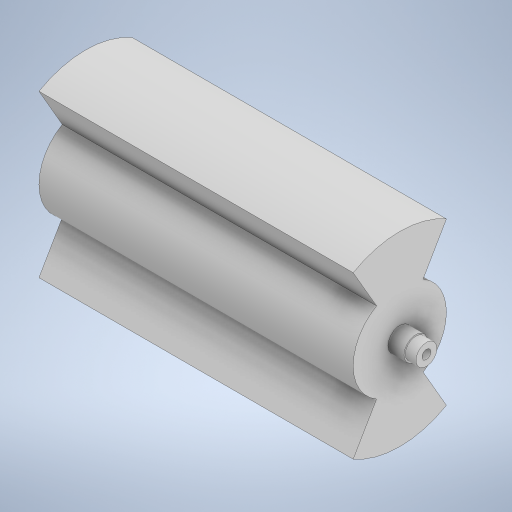
# Autodesk Inventor part: newDrum
Saved by Autodesk Inventor 2024.2 (Build 282272000, 272)
## iProperties
Created: 2024-02-27
Part Number: newDrum
Material: Generic
Document SubType Name: Modeling
Designer: jerem
Density: 1 g/cm^3
Appearance: Default
Author: jerem
## iProperties of the stored document newDrum_3DPrint.ipt
Created: 2024-02-27
Part Number: newDrum_3DPrint
Material: Generic
Document SubType Name: Modeling
Designer: jerem
Density: 1 g/cm^3
Appearance: Default
Author: jerem
Autodesk Inventor part; units mm, degrees
ref_plane "YZ Plane" through (0, 0, 0) normal (1, 0, 0) x (0, 1, 0)
ref_plane "XZ Plane" through (0, 0, 0) normal (0, 1, 0) x (-1, 0, 0)
ref_plane "XY Plane" through (0, 0, 0) normal (0, 0, 1) x (1, 0, 0)
sketch "Sketch1" plane through (0, 0, 0) normal (1, 0, 0) x (0, 1, 0)
  circle A0 centre (0, 0) radius 17.5
  dimension "d1" = 35
  constraints: 1 centre point
  measures "d1" diameter of A0
extrude "Extrusion1" add sketch "Sketch1" along normal blind 118
sketch "Sketch2" plane through (0, 0, 0) normal (-1, 0, 0) x (0, 0, 1)
  circle A0 centre (0, 0) radius 13.9
  dimension "d4" = 27.8
  constraints: 1 centre point, 1 coincident
  measures "d4" diameter of A0
extrude "Extrusion2" cut sketch "Sketch2" against normal blind 16
sketch "Sketch3" plane through (16, 0, 0) normal (-1, 0, 0) x (0, 0, 1)
  circle A0 centre (0, 0) radius 4.85
  dimension "d7" = 9.7
  constraints: 1 centre point, 1 coincident
  measures "d7" diameter of A0
extrude "Extrusion3" cut sketch "Sketch3" against normal blind 4.2
sketch "Sketch4" plane through (20.2, 0, 0) normal (-1, 0, 0) x (0, 0, 1)
  circle A0 centre (0, 0) radius 1.7
  dimension "d10" = 3.4
  constraints: 1 centre point, 1 coincident
  measures "d10" diameter of A0
extrude "Extrusion4" cut sketch "Sketch4" against normal blind 10
sketch "Sketch9" plane through (0, 0, 0) normal (1, 0, 0) x (0, 1, 0)
  circle A0 centre (0, 0) radius 1.7 construction
  circle A1 centre (0, 0) radius 35 construction
  line L0 (-35, 0) -> (-17.5, 0)
  circle A2 centre (0, 0) radius 17.5 construction
  line L1 (-15.1554, 8.75) -> (-30.3109, 17.5)
  arc A3 (-30.3109, 17.5) -> (-35, 0) centre (0, 0) ccw
  arc A4 (-15.1554, 8.75) -> (-17.5, 0) centre (0, 0) ccw
  dimension "d32" = 70
  dimension "d33" = 30
  constraints: 8 point on circle, 4 end point, 3 centre point, 3 line through centre, 2 concentric, 1 coincident, 1 horizontal
  measures "d32" diameter of A1
  measures "d33" angle of L1 L0
extrude "Extrusion8" add sketch "Sketch9" along normal up to surface (118 mm away)
sketch "Sketch10" plane through (118, 0, 0) normal (1, 0, 0) x (0, 0, -1)
  circle A0 centre (0, 0) radius 1.7 projected
  circle A1 centre (0, 0) radius 3.925
  dimension "d36" = 7.85
  constraints: 1 centre point, 1 coincident
  measures "d36" diameter of A1
extrude "Extrusion9" add sketch "Sketch10" along normal blind 10
sketch "Sketch12" plane through (118, 0, 0) normal (1, 0, 0) x (0, 0, -1)
  circle A0 centre (0, 0) radius 4.445
  dimension "d42" = 8.89
  constraints: 1 centre point, 1 coincident
  measures "d42" diameter of A0
extrude "Extrusion11" add sketch "Sketch12" along normal blind 6
sketch "Sketch11" plane through (118, 0, 0) normal (1, 0, 0) x (0, 0, -1)
  circle A0 centre (0, 0) radius 4.85 projected
  circle A1 centre (0, 0) radius 1.7
  constraints: 1 centre point, 1 coincident
extrude "Extrusion10" cut sketch "Sketch11" against normal blind 20 from surface at 10 contours A1
mirror "Mirror1" about plane through (0, 0, 0) normal (0, 0, 1) of "Extrusion8"
mirror "Mirror2" about plane through (0, 0, 0) normal (0, 1, 0) of "Extrusion8", "Mirror1"
body "Solid1"
